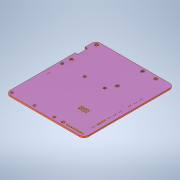
# Autodesk Inventor part: buoy_pcb
Saved by Autodesk Inventor 2020.2 (Build 242310000, 310)
## iProperties
Created: 2020-04-10
Part Number: buoy_pcb
Material: Phenolic Resin
Document SubType Name: Modeling
Designer: agmlego
Mass: 20.3052 g
Surface Area: 193.493 cm^2
Volume: 14.7139 cm^3
Density: 1.38 g/cm^3
Appearance: Smooth - Light Orange
Author: agmlego
Autodesk Inventor part; units mm, degrees
ref_plane "YZ Plane" through (0, 0, 0) normal (1, 0, 0) x (0, 1, 0)
ref_plane "XZ Plane" through (0, 0, 0) normal (0, 1, 0) x (-1, 0, 0)
ref_plane "XY Plane" through (0, 0, 0) normal (0, 0, 1) x (1, 0, 0)
sketch "Sketch1" plane through (0, 0, 0) normal (0, 1, 0) x (-1, 0, 0)
  line L0 (0, 0) -> (90, 0)
  line L1 (90, -104) -> (0, -104)
  line L2 (0, -104) -> (0, 0)
  line L3 (90, -91) -> (87, -91)
  line L4 (87, -91) -> (87, -80)
  line L5 (87, -80) -> (90, -80)
  line L6 (90, 0) -> (90, -80)
  line L7 (90, -91) -> (90, -104)
  dimension "d0" = 104
  dimension "d1" = 90
  dimension "d32" = 11
  dimension "d33" = 3
  dimension "d35" = 80
  constraints: 16 end point, 5 perpendicular, 3 parallel, 2 horizontal, 1 coincident, 1 collinear
  measures "d0" distance of L0.end L1.start
  measures "d1" distance of L0.start L0.end
  measures "d32" distance of L3.end L4.end
  measures "d33" distance of L4.end L5.end
  measures "d35" distance between parallel lines of L0 L5
extrude "PCB" add sketch "Sketch1" along normal blind 1.6
sketch "Sketch2" plane through (0, 1.6, 0) normal (0, 1, 0) x (1, 0, 0)
  line L0 (-86.55, 3.55) -> (-86.55, 61.55) construction
  line L1 (-86.55, 3.55) -> (-60.56, 3.55) construction
  line L2 (-60.56, 3.55) -> (-37.56, 3.55) construction
  line L3 (-37.56, 3.55) -> (-37.56, 61.55) construction
  line L4 (-37.56, 61.55) -> (-60.56, 61.55) construction
  line L5 (-60.56, 61.55) -> (-60.56, 3.55) construction
  line L6 (-60.56, 61.55) -> (-86.55, 61.55) construction
  line L7 (-60.56, 0.05) -> (-37.56, 0.05) construction
  line L8 (-34.06, 3.55) -> (-34.06, 61.55) construction
  line L9 (-37.56, 65.05) -> (-60.56, 65.05) construction
  line L10 (-64.06, 61.55) -> (-64.06, 3.55) construction
  arc A0 (-64.06, 3.55) -> (-60.56, 0.05) centre (-60.56, 3.55) ccw construction
  arc A1 (-37.56, 0.05) -> (-34.06, 3.55) centre (-37.56, 3.55) ccw construction
  arc A2 (-34.06, 61.55) -> (-37.56, 65.05) centre (-37.56, 61.55) ccw construction
  arc A3 (-60.56, 65.05) -> (-64.06, 61.55) centre (-60.56, 61.55) ccw construction
  point P0 (0, 0)
  point P1 (-64.06, 0.05)
  point P2 (-34.06, 65.05)
  point P3 (-34.06, 0.05)
  dimension "d4" = 86.55
  dimension "d5" = 3.55
  dimension "d6" = 61.55
  dimension "d7" = 23
  dimension "d8" = 30
  dimension "d9" = 65
  dimension "d10" = 3.5
  dimension "d11" = 64.06
  constraints: 22 end point, 8 point on circle, 8 tangent, 6 point on line, 4 centre point, 3 equal radius, 3 perpendicular, 2 collinear, 2 horizontal, 2 parallel, 2 vertical, 1 coincident
  measures "d4" horizontal distance of point (0, 0) L0.start
  measures "d5" vertical distance of point (0, 0) L0.start
  measures "d6" vertical distance of point (0, 0) L0.end
  measures "d7" distance of L1.end L2.end
  measures "d8" distance of point (-64.06, 0.05) point (-34.06, 0.05)
  measures "d9" distance of point (-34.06, 0.05) point (-34.06, 65.05)
  measures "d10" radius of A0
  measures "d11" distance from line of point (0, 0) L10
hole "Pi and HAT Mounting" at (-86.55, 1.6, -3.55) at (-60.56, 1.6, -3.55) at (-37.56, 1.6, -3.55) at (-37.56, 1.6, -61.55) at (-60.56, 1.6, -61.55) at (-86.55, 1.6, -61.55) direction (0, -1, 0) diameter 2.75 end through all start extended yes
sketch "Sketch3" plane through (0, 1.6, 0) normal (0, 1, 0) x (1, 0, 0)
  line L0 (-89.37, 67.02) -> (-28.37, 67.02) construction
  line L1 (-28.37, 67.02) -> (-28.37, 104.02) construction
  line L2 (-28.37, 104.02) -> (-89.37, 104.02) construction
  line L3 (-89.37, 104.02) -> (-89.37, 67.02) construction
  circle A0 centre (-32.3213, 70.9713) radius 3.9513 construction
  circle A1 centre (-32.3213, 100.0687) radius 3.9513 construction
  circle A2 centre (-85.37, 100.02) radius 4 construction
  circle A3 centre (-85.37, 71.02) radius 4 construction
  point P0 (0, 0)
  dimension "d19" = 8
  dimension "d20" = 61
  dimension "d21" = 37
  dimension "d22" = 104.02
  dimension "d23" = 28.37
  constraints: 8 end point, 8 tangent, 4 centre point, 4 coincident, 2 equal radius, 2 parallel, 1 horizontal, 1 perpendicular
  measures "d19" diameter of A3
  measures "d20" distance of L0.start L0.end
  measures "d21" distance of L0.end L1.end
  measures "d22" distance from line of point (0, 0) L2
  measures "d23" distance from line of point (0, 0) L1
hole "Xtend Mounting" at (-85.37, 1.6, -71.02) at (-85.37, 1.6, -100.02) at (-32.3213, 1.6, -100.0687) at (-32.3213, 1.6, -70.9713) direction (0, -1, 0) diameter 3.3 end through all start extended yes
fillet "Corner Break" radius 5 4 edges at (-90, 0.8, 0) (0, 0.8, 0) (0, 0.8, -104) (-90, 0.8, -104)
fillet "Slot Corner Break" radius 0.254 4 edges at (-90, 0.8, -91) (-87, 0.8, -91) (-87, 0.8, -80) (-90, 0.8, -80)
sketch "Sketch26" plane through (0, 1.6, 0) normal (0, 1, 0) x (1, 0, 0)
  circle A0 centre (-86.55, 3.55) radius 1.375 construction
  circle A1 centre (-85.37, 100.02) radius 1.65 construction
  circle A2 centre (-32.3213, 100.0687) radius 1.65 construction
  circle A3 centre (-37.56, 3.55) radius 1.375 construction
  line L0 (-86.55, 3.55) -> (-27.56, 3.55) construction
  line L1 (-85.37, 100.02) -> (-17.3213, 100.0825) construction
  line L2 (0, 5) -> (0, 99) construction
  line L3 (-85, 0) -> (-5, 0) construction
  point P0 (0, 0)
  dimension "d97" = 10
  dimension "d98" = 15
  dimension "d99" = 17.3213
  dimension "d100" = 100.0825
  dimension "d101" = 3.55
  dimension "d102" = 27.56
  constraints: 4 end point, 2 point on line
  measures "d97" distance of L0.end A3.centre
  measures "d98" distance of A2.centre L1.end
  measures "d99" distance from line of L2 L1.end
  measures "d100" distance from line of L3 L1.end
  measures "d101" distance from line of L3 L0.end
  measures "d102" distance from line of L2 L0.end
hole "Mounting" at (-27.56, 1.6, -3.55) at (-17.3213, 1.6, -100.0825) direction (0, -1, 0) diameter 3.3 end through all start extended yes
sketch "Sketch4" plane through (0, 1.6, 0) normal (0, 1, 0) x (1, 0, 0)
  line L0 (-5.21, 16.91) -> (-5.21, 14.91) construction
  line L1 (-5.21, 35.21) -> (-5.21, 33.21) construction
  line L2 (-5.21, 41.56) -> (-5.21, 39.56) construction
  line L3 (-5.21, 47.86) -> (-5.21, 45.86) construction
  line L4 (-84.74, 43.08) -> (-84.74, 45.08) construction
  line L5 (-5.21, 59) -> (-5.21, 57) construction
  line L6 (-5.21, 65.62) -> (-5.21, 63.62) construction
  line L7 (-5.21, 71.97) -> (-5.21, 69.97) construction
  line L8 (-5.21, 15.91) -> (-2.4814, 15.91) construction
  line L9 (-5.21, 34.21) -> (-2.0979, 34.21) construction
  line L10 (-5.21, 40.56) -> (-2.0979, 40.56) construction
  line L11 (-5.21, 46.86) -> (-2.0979, 46.86) construction
  line L12 (-5.21, 58) -> (-2.2755, 58) construction
  line L13 (-5.21, 64.62) -> (-2.3783, 64.62) construction
  line L14 (-5.21, 70.97) -> (-2.2755, 70.97) construction
  line L15 (-84.74, 44.08) -> (-88.2856, 44.08) construction
  point P0 (0, 0)
  dimension "d37" = 2
  dimension "d38" = 15.91
  dimension "d39" = 70.97
  dimension "d40" = 64.62
  dimension "d41" = 58
  dimension "d42" = 46.86
  dimension "d43" = 40.56
  dimension "d44" = 34.21
  dimension "d45" = 5.21
  dimension "d46" = 44.08
  dimension "d47" = 84.74
  constraints: 32 end point, 8 horizontal, 8 midpoint, 8 vertical, 7 equal length, 6 collinear
  measures "d37" distance of L0.start L0.end
  measures "d38" distance from line of point (0, 0) L8
  measures "d39" distance from line of L14 point (0, 0)
  measures "d40" distance from line of point (0, 0) L13
  measures "d41" distance from line of point (0, 0) L12
  measures "d42" distance from line of L11 point (0, 0)
  measures "d43" distance from line of L10 point (0, 0)
  measures "d44" distance from line of L9 point (0, 0)
  measures "d45" distance from line of L0 point (0, 0)
  measures "d46" distance from line of L15 point (0, 0)
  measures "d47" distance from line of point (0, 0) L4
hole "JST-PH-2" at (-5.21, 1.6, -16.91) at (-5.21, 1.6, -14.91) at (-5.21, 1.6, -35.21) at (-5.21, 1.6, -33.21) at (-5.21, 1.6, -41.56) at (-5.21, 1.6, -39.56) at (-5.21, 1.6, -47.86) at (-5.21, 1.6, -45.86) at (-84.74, 1.6, -43.08) at (-84.74, 1.6, -45.08) at (-5.21, 1.6, -59) at (-5.21, 1.6, -57) at (-5.21, 1.6, -65.62) at (-5.21, 1.6, -63.62) at (-5.21, 1.6, -71.97) at (-5.21, 1.6, -69.97) direction (0, -1, 0) diameter 0.7 end through all start extended yes
sketch "Sketch5" plane through (0, 1.6, 0) normal (0, 1, 0) x (1, 0, 0)
  line L0 (-85, 0) -> (-5, 0) construction
  line L1 (0, 5) -> (0, 99) construction
  point P0 (0, 0)
  point P1 (-22.39, 3.03)
  point P2 (-19.85, 3.03)
  point P3 (-17.31, 3.03)
  point P4 (-14.77, 3.03)
  point P5 (-12.23, 3.03)
  point P6 (-9.69, 3.03)
  point P7 (-7.15, 3.03)
  point P8 (-4.61, 3.03)
  point P9 (-5.03, 21.18)
  point P10 (-5.03, 23.72)
  point P11 (-5.03, 26.26)
  point P12 (-5.03, 28.8)
  point P13 (-31.85, 26.53)
  point P14 (-29.31, 26.53)
  point P15 (-26.77, 26.53)
  point P16 (-24.23, 26.53)
  point P17 (-31.85, 29.38)
  point P18 (-29.31, 29.38)
  point P19 (-26.77, 29.38)
  point P20 (-24.23, 29.38)
  dimension "d57" = 2.54
  dimension "d62" = 3.03
  dimension "d63" = 22.39
  dimension "d66" = 2.54
  dimension "d71" = 21.18
  dimension "d72" = 5.03
  dimension "d75" = 2.54
  dimension "d82" = 2.54
  dimension "d87" = 31.85
  dimension "d88" = 26.53
  dimension "d89" = 29.38
  constraints: 3 horizontal, 1 vertical, 1 vertical alignment, 16 other
  measures "d57" distance of point (-22.39, 3.03) point (-19.85, 3.03)
  measures "d62" distance from line of L0 point (-22.39, 3.03)
  measures "d63" distance from line of L1 point (-22.39, 3.03)
  measures "d66" distance of point (-5.03, 21.18) point (-5.03, 23.72)
  measures "d71" vertical distance of point (0, 0) point (-5.03, 21.18)
  measures "d72" distance from line of L1 point (-5.03, 21.18)
  measures "d75" distance of point (-31.85, 26.53) point (-29.31, 26.53)
  measures "d82" distance of point (-31.85, 29.38) point (-29.31, 29.38)
  measures "d87" horizontal distance of point (0, 0) point (-31.85, 26.53)
  measures "d88" vertical distance of point (0, 0) point (-31.85, 26.53)
  measures "d89" vertical distance of point (0, 0) point (-31.85, 29.38)
hole "0.1\" Pin Headers" at (-22.39, 1.6, -3.03) at (-19.85, 1.6, -3.03) at (-17.31, 1.6, -3.03) at (-14.77, 1.6, -3.03) at (-12.23, 1.6, -3.03) at (-9.69, 1.6, -3.03) at (-7.15, 1.6, -3.03) at (-4.61, 1.6, -3.03) at (-5.03, 1.6, -21.18) at (-5.03, 1.6, -23.72) at (-5.03, 1.6, -26.26) at (-5.03, 1.6, -28.8) at (-31.85, 1.6, -26.53) at (-29.31, 1.6, -26.53) at (-26.77, 1.6, -26.53) at (-24.23, 1.6, -26.53) at (-31.85, 1.6, -29.38) at (-29.31, 1.6, -29.38) at (-26.77, 1.6, -29.38) at (-24.23, 1.6, -29.38) direction (0, -1, 0) diameter 1.016 end through all start extended yes
sketch "Sketch6" plane through (0, 1.6, 0) normal (0, 1, 0) x (1, 0, 0)
  circle A0 centre (-22.39, 3.03) radius 0.508 construction
sketch "Sketch7" plane through (0, 1.6, 0) normal (0, 1, 0) x (1, 0, 0)
  circle A0 centre (-19.85, 3.03) radius 0.508 construction
sketch "Sketch8" plane through (0, 1.6, 0) normal (0, 1, 0) x (1, 0, 0)
  circle A0 centre (-17.31, 3.03) radius 0.508 construction
sketch "Sketch9" plane through (0, 1.6, 0) normal (0, 1, 0) x (1, 0, 0)
  circle A0 centre (-14.77, 3.03) radius 0.508 construction
sketch "Sketch10" plane through (0, 1.6, 0) normal (0, 1, 0) x (1, 0, 0)
  circle A0 centre (-12.23, 3.03) radius 0.508 construction
sketch "Sketch11" plane through (0, 1.6, 0) normal (0, 1, 0) x (1, 0, 0)
  circle A0 centre (-9.69, 3.03) radius 0.508 construction
sketch "Sketch12" plane through (0, 1.6, 0) normal (0, 1, 0) x (1, 0, 0)
  circle A0 centre (-7.15, 3.03) radius 0.508 construction
sketch "Sketch13" plane through (0, 1.6, 0) normal (0, 1, 0) x (1, 0, 0)
  circle A0 centre (-4.61, 3.03) radius 0.508 construction
sketch "Sketch14" plane through (0, 1.6, 0) normal (0, 1, 0) x (1, 0, 0)
  circle A0 centre (-5.03, 21.18) radius 0.508 construction
sketch "Sketch15" plane through (0, 1.6, 0) normal (0, 1, 0) x (1, 0, 0)
  circle A0 centre (-5.03, 23.72) radius 0.508 construction
sketch "Sketch16" plane through (0, 1.6, 0) normal (0, 1, 0) x (1, 0, 0)
  circle A0 centre (-5.03, 26.26) radius 0.508 construction
sketch "Sketch17" plane through (0, 1.6, 0) normal (0, 1, 0) x (1, 0, 0)
  circle A0 centre (-5.03, 28.8) radius 0.508 construction
sketch "Sketch18" plane through (0, 1.6, 0) normal (0, 1, 0) x (1, 0, 0)
  circle A0 centre (-31.85, 26.53) radius 0.508 construction
sketch "Sketch19" plane through (0, 1.6, 0) normal (0, 1, 0) x (1, 0, 0)
  circle A0 centre (-29.31, 26.53) radius 0.508 construction
sketch "Sketch20" plane through (0, 1.6, 0) normal (0, 1, 0) x (1, 0, 0)
  circle A0 centre (-26.77, 26.53) radius 0.508 construction
sketch "Sketch21" plane through (0, 1.6, 0) normal (0, 1, 0) x (1, 0, 0)
  circle A0 centre (-24.23, 26.53) radius 0.508 construction
sketch "Sketch22" plane through (0, 1.6, 0) normal (0, 1, 0) x (1, 0, 0)
  circle A0 centre (-31.85, 29.38) radius 0.508 construction
sketch "Sketch23" plane through (0, 1.6, 0) normal (0, 1, 0) x (1, 0, 0)
  circle A0 centre (-29.31, 29.38) radius 0.508 construction
sketch "Sketch24" plane through (0, 1.6, 0) normal (0, 1, 0) x (1, 0, 0)
  circle A0 centre (-26.77, 29.38) radius 0.508 construction
sketch "Sketch25" plane through (0, 1.6, 0) normal (0, 1, 0) x (1, 0, 0)
  circle A0 centre (-24.23, 29.38) radius 0.508 construction
body "Solid1"
